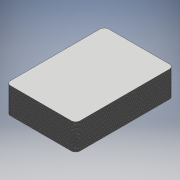
# Autodesk Inventor part: Game_CardDeck0.25
Saved by Autodesk Inventor 2018 (Build 220112000, 112)
## iProperties
Created: 2021-04-21
Part Number: Game_CardDeck0.25
Material: Generic
Document SubType Name: Modeling
Designer: Bradley
Density: 1 g/cm^3
Appearance: Default
Author: Bradley
Autodesk Inventor part; units mm, degrees
ref_plane "YZ Plane" through (0, 0, 0) normal (1, 0, 0) x (0, 1, 0)
ref_plane "XZ Plane" through (0, 0, 0) normal (0, 1, 0) x (-1, 0, 0)
ref_plane "XY Plane" through (0, 0, 0) normal (0, 0, 1) x (1, 0, 0)
sketch "Sketch1" plane through (0, 0, 0) normal (0, 0, 1) x (1, 0, 0)
  line L0 (-27.5, -44.5) -> (27.5, -44.5)
  line L1 (31.5, -40.5) -> (31.5, 40.5)
  line L2 (27.5, 44.5) -> (-27.5, 44.5)
  line L3 (-31.5, 40.5) -> (-31.5, -40.5)
  line L4 (-31.5, -44.5) -> (31.5, 44.5) construction
  line L5 (31.5, -44.5) -> (-31.5, 44.5) construction
  arc A0 (31.5, 40.5) -> (27.5, 44.5) centre (27.5, 40.5) ccw
  arc A1 (27.5, -44.5) -> (31.5, -40.5) centre (27.5, -40.5) ccw
  arc A2 (-31.5, -40.5) -> (-27.5, -44.5) centre (-27.5, -40.5) ccw
  arc A3 (-27.5, 44.5) -> (-31.5, 40.5) centre (-27.5, 40.5) ccw
  point P0 (0, 0)
  dimension "d0" = 63
  dimension "d1" = 89
  dimension "d2" = 4
  constraints: 12 end point, 8 point on circle, 8 point on line, 8 tangent, 4 centre point, 3 equal radius, 2 midpoint, 2 parallel, 1 horizontal, 1 perpendicular
  measures "d0" distance of L5.end L4.end
  measures "d1" distance of L4.end L5.start
  measures "d2" radius of A0
extrude "Extrusion1" add sketch "Sketch1" along normal mid plane 0.27
pattern_linear "Rectangular Pattern1" count 83 spacing 0.2858 along (0, 0, 1) of "Extrusion1"
body "Solid1"
